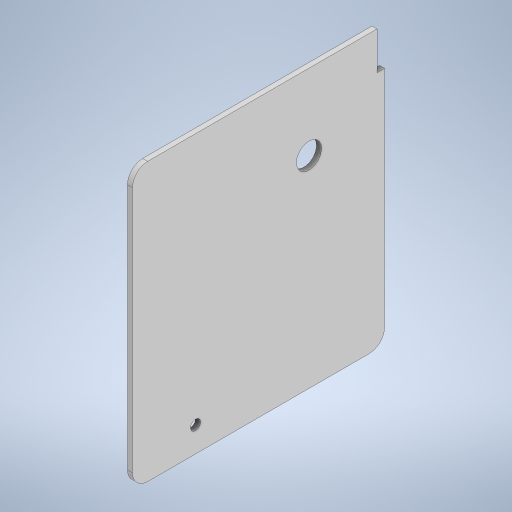
# Autodesk Inventor part: WI-Cover
Saved by Autodesk Inventor 2024.3 (Build 283343000, 343)
## iProperties
Created: 2025-06-26
Part Number: WI-Cover
Material: Generic
Document SubType Name: Sheet Metal
Designer: ajclo
Density: 1 g/cm^3
Sheet Metal Rule: Default_mm
Appearance: Default
Author: ajclo
Autodesk Inventor part; units mm, degrees
ref_plane "YZ Plane" through (0, 0, 0) normal (1, 0, 0) x (0, 1, 0)
ref_plane "XZ Plane" through (0, 0, 0) normal (0, 1, 0) x (-1, 0, 0)
ref_plane "XY Plane" through (0, 0, 0) normal (0, 0, 1) x (1, 0, 0)
sketch "Sketch1" plane through (0, 0, 0) normal (1, 0, 0) x (0, 1, 0)
  line L0 (0, 0) -> (110, 0)
  line L1 (110, 0) -> (110, -100)
  line L2 (110, -100) -> (0, -100)
  line L3 (0, -100) -> (0, 0)
  line L4 (110, -97) -> (95, -97)
  line L5 (95, -97) -> (95, -100)
  line L6 (95, -100) -> (110, -100)
  line L7 (110, -100) -> (110, -97)
  circle A0 centre (10, -25) radius 2
  circle A1 centre (80, -70) radius 5
  point P0 (102.5, -100)
  point P1 (102.5, -97)
  point P2 (110, -98.5)
  point P3 (95, -98.5)
  dimension "d0" = 110
  dimension "d1" = 100
  dimension "d2" = 3
  dimension "d3" = 15
  dimension "d4" = 4
  dimension "d5" = 10
  dimension "d6" = 25
  dimension "d9" = 10
  dimension "d10" = 30
  dimension "d11" = 30
  measures "d0" distance of L1.end L2.end
  measures "d1" distance of L0.end L1.end
  measures "d2" distance of point (102.5, -100) point (102.5, -97)
  measures "d3" distance of point (110, -98.5) point (95, -98.5)
  measures "d4" diameter of A0
  measures "d5" distance from line of L3 A0.centre
  measures "d6" distance from line of L0 A0.centre
  measures "d9" diameter of A1
  measures "d10" distance from line of L1 A1.centre
  measures "d11" distance from line of L2 A1.centre
extrude "Plate2" add sketch "Sketch1" along normal blind 2 contours L0 L1 L4 L5 L2 L3
fillet "Corner Round2" radius 6 3 edges at (1, 110, 0) (1, 0, 0) (1, 0, -100)
equation "\"d12\" = Thickness"
equation "\"BendRadius\" = Thickness"
equation "\"BendReliefWidth\" = Thickness"
equation "\"BendReliefDepth\" = 0.5 * Thickness"
equation "\"CornerReliefSize\" = 4 * Thickness"
equation "\"MinimumRemnant\" = 2 * Thickness"
equation "\"TransitionRadius\" = BendRadius"
equation "\"JacobiRadiusSize\" = BendRadius"
equation "\"GapSize\" = Thickness"
equation "\"Thickness\" = 2"
body "Solid2"
